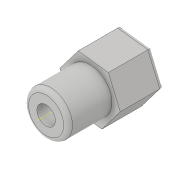
# Autodesk Inventor part: Suction_electrode_cap
Saved by Autodesk Inventor 2020 (Build 240168000, 168)
## iProperties
Created: 2020-05-16
Part Number: Suction_electrode_cap
Material: Generic
Document SubType Name: Modeling
Designer: Huai-Ti Lin
Density: 1 g/cm^3
Appearance: Default
Author: Huai-Ti Lin
Autodesk Inventor part; units mm, degrees
ref_plane "YZ Plane" through (0, 0, 0) normal (1, 0, 0) x (0, 1, 0)
ref_plane "XZ Plane" through (0, 0, 0) normal (0, 1, 0) x (-1, 0, 0)
ref_plane "XY Plane" through (0, 0, 0) normal (0, 0, 1) x (1, 0, 0)
sketch "Sketch1" plane through (0, 0, 0) normal (0, 1, 0) x (-1, 0, 0)
  line L0 (-1.05, 6.1643) -> (-2.5, 6.1643)
  line L1 (-2.5, 6.1643) -> (-2.5, 1.1643)
  line L2 (-2.5, 1.1643) -> (-3.5, 1.1643)
  line L3 (-3.5, 1.1643) -> (-3.5, -3.8357)
  line L4 (-3.5, -3.8357) -> (-1.05, -3.8357)
  line L5 (0, -5.8357) -> (0, 8.1643) projected
  line L6 (-1.05, 6.1643) -> (-1.05, -3.8357)
  point P0 (0, 0)
  dimension "d0" = 5
  dimension "d1" = 5
  dimension "d3" = 1.05
  dimension "d4" = 2.5
  dimension "d5" = 3.5
  constraints: 13 end point, 4 perpendicular, 1 horizontal
  measures "d0" distance of L2.end L3.end
  measures "d1" distance between parallel lines of L2 L0
  measures "d3" distance between parallel lines of L5 L6
  measures "d4" distance between parallel lines of L5 L1
  measures "d5" distance between parallel lines of L5 L3
revolve "Revolution1" add sketch "Sketch1" angle 360 about axis through (0, 0, -10) along (0, 0, 1)
sketch "Sketch2" plane through (0, 0, -3.8357) normal (0, 0, -1) x (-1, 0, 0)
  circle A0 centre (0, 0) radius 3.5 projected
  line L0 (1.3478, 3.1911) -> (3.4375, 0.4283)
  line L1 (3.4375, 0.4283) -> (2.0897, -2.7628)
  line L2 (2.0897, -2.7628) -> (-1.3478, -3.1911)
  line L3 (-1.3478, -3.1911) -> (-3.4375, -0.4283)
  line L4 (-3.4375, -0.4283) -> (-2.0897, 2.7628)
  line L5 (-2.0897, 2.7628) -> (1.3478, 3.1911)
  circle A1 centre (0, 0) radius 5.601
  dimension "d8" = 7
  dimension "d10" = 6
  constraints: 12 end point, 1 centre point, 1 coincident, 13 other
  measures "d8" diameter of A0
  measures "d10" distance between parallel lines of L2 L5
extrude "Extrusion1" cut sketch "Sketch2" against normal blind 10 contours A0 | A1
fillet "Fillet2" radius 0.5 7 edges at (-2.7636, -1.1672, -3.8357) (-2.3927, 1.8097, -3.8357) (0.3709, 2.977, -3.8357) (2.7636, 1.1672, -3.8357) (2.3927, -1.8097, -3.8357) (-0.3709, -2.977, -3.8357) (-2.5, 0, 6.1643)
body "Solid1"
